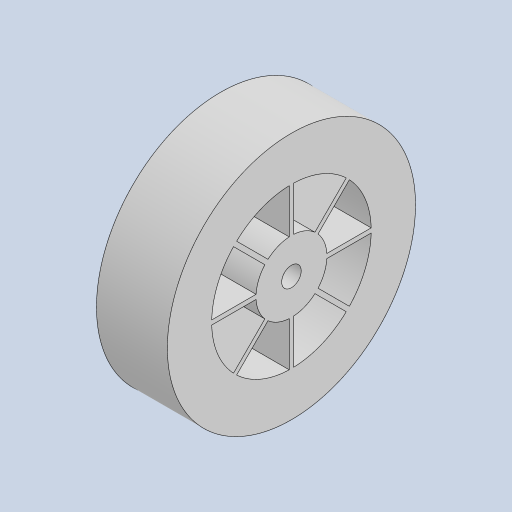
# Autodesk Inventor part: wheel
Saved by Autodesk Inventor 2023 (Build 270158000, 158)
## iProperties
Created: 2022-06-17
Part Number: wheel
Material: 一般
Document SubType Name: Modeling
Designer: legot
Density: 1 g/cm^3
Appearance: 既定
Author: legot
Autodesk Inventor part; units mm, degrees
ref_plane "YZ Plane" through (0, 0, 0) normal (1, 0, 0) x (0, 1, 0)
ref_plane "XZ Plane" through (0, 0, 0) normal (0, 1, 0) x (-1, 0, 0)
ref_plane "XY Plane" through (0, 0, 0) normal (0, 0, 1) x (1, 0, 0)
sketch "スケッチ1" plane through (0, 0, 0) normal (1, 0, 0) x (0, 1, 0)
  circle A0 centre (0, 0) radius 14
  dimension "d0" = 28
  constraints: 1 centre point, 1 coincident
  measures "d0" diameter of A0
extrude "押し出し1" add sketch "スケッチ1" along normal mid plane 8
sketch "スケッチ2" plane through (4, 0, 0) normal (1, 0, 0) x (0, 0, -1)
  circle A0 centre (0, 0) radius 14 projected
  circle A1 centre (0, 0) radius 4
  circle A2 centre (0, 0) radius 9
  line L0 (0.25, 3.9922) -> (0.25, 8.9965)
  line L1 (-0.25, 3.9922) -> (-0.25, 8.9965)
  line L2 (2.6461, 2.9997) -> (6.1847, 6.5383)
  line L3 (2.9997, 2.6461) -> (6.5383, 6.1847)
  point P0 (-0.25, 6.4944)
  point P1 (0.25, 6.4944)
  dimension "d3" = 8
  dimension "d4" = 18
  dimension "d5" = 0.5
  dimension "d6" = 0.5
  dimension "d7" = 45
  constraints: 8 end point, 8 point on circle, 3 parallel, 2 centre point, 2 midpoint, 2 vertical
  measures "d3" diameter of A1
  measures "d4" diameter of A2
  measures "d5" distance of point (-0.25, 6.494) point (0.25, 6.494)
  measures "d6" distance between parallel lines of L2 L3
  measures "d7" angle of L0 L2
extrude "押し出し2" cut sketch "スケッチ2" against normal through all contours A1 L0 A2 L2
pattern_circular "円形状パターン1" count 8 over 360 about axis through (0, 0, 0) along (1, 0, 0) of "押し出し2"
sketch "スケッチ3" plane through (4, 0, 0) normal (1, 0, 0) x (0, 0, -1)
  circle A0 centre (0, 0) radius 14 projected
  constraints: 1 coincident
hole "穴1" at (4, 0, 0) direction (-1, 0, 0) diameter 2.2 end through all
equation "\"d6\" = d5"
